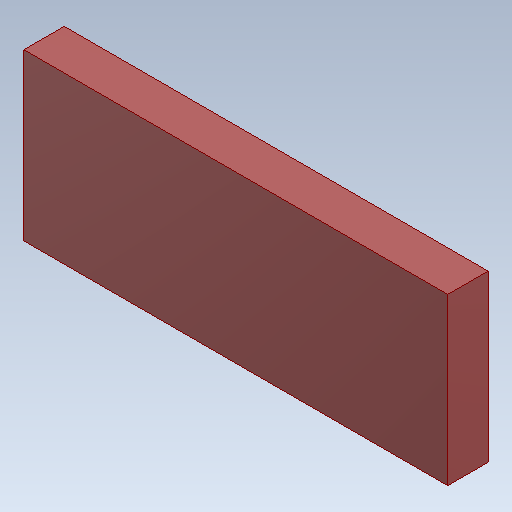
# Autodesk Inventor part: 53261-04
Saved by Autodesk Inventor 2020 (Build 240168000, 168)
## iProperties
Created: 2019-05-24
Part Number: 53261-04
Material: Generic
Document SubType Name: Modeling
Designer: psrob
Density: 1 g/cm^3
Appearance: 53261-04, 53261-04
Author: psrob
Autodesk Inventor part; units mm, degrees
ref_plane "YZ Plane" through (0, 0, 0) normal (1, 0, 0) x (0, 1, 0)
ref_plane "XZ Plane" through (0, 0, 0) normal (0, 1, 0) x (-1, 0, 0)
ref_plane "XY Plane" through (0, 0, 0) normal (0, 0, 1) x (1, 0, 0)
sketch "53261-04, 53261-04_22" plane through (0, 0, 0) normal (0, 0, 1) x (1, 0, 0)
  line L0 (-5.25, 2.625) -> (5.25, 2.625)
  line L1 (5.25, 2.625) -> (5.25, -1.4766)
  line L2 (5.25, -1.4766) -> (-5.25, -1.4766)
  line L3 (-5.25, -1.4766) -> (-5.25, 2.625)
  constraints: 8 end point
extrude "Extrusion1" add sketch "53261-04, 53261-04_22" along normal blind 1
body "Solid1"
